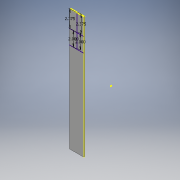
# Autodesk Inventor part: long metal piece 2x17
Saved by Autodesk Inventor 2017 (Build 210142000, 142)
## iProperties
Created: 2017-03-02
Part Number: long metal piece 2x17
Material: Generic
Document SubType Name: Modeling
Designer: Jess
Density: 1 g/cm^3
Appearance: Default
Author: Jess
Autodesk Inventor part; units mm, degrees
ref_plane "YZ Plane" through (0, 0, 0) normal (1, 0, 0) x (0, 1, 0)
ref_plane "XZ Plane" through (0, 0, 0) normal (0, 1, 0) x (-1, 0, 0)
ref_plane "XY Plane" through (0, 0, 0) normal (0, 0, 1) x (1, 0, 0)
sketch "Sketch1" plane through (0, 0, 0) normal (0, 0, 1) x (1, 0, 0)
  line L0 (-144.6628, 165.0655) -> (-93.8628, 165.0655)
  line L1 (-93.8628, 165.0655) -> (-93.8628, -263.5595)
  line L2 (-93.8628, -263.5595) -> (-144.6628, -263.5595)
  line L3 (-144.6628, -263.5595) -> (-144.6628, 165.0655)
  line L4 (-119.2628, 165.0655) -> (-119.2628, 104.7405)
  line L5 (-119.2628, 104.7405) -> (-144.6628, 104.7405)
  line L6 (-93.8628, 104.7405) -> (-119.2628, 104.7405)
  point P0 (0, 0)
  dimension "d0" = 50.8
  dimension "d1" = 428.625
  dimension "d4" = 60.325
  constraints: 14 end point, 3 perpendicular, 3 point on line, 2 parallel, 1 horizontal, 1 midpoint, 1 vertical
  measures "d0" distance of L1.end L2.end
  measures "d1" distance of L0.end L1.end
  measures "d4" distance of L4.start L4.end
extrude "Extrusion1" add sketch "Sketch1" along normal blind 3.175
sketch "Sketch2" plane through (0, 0, 3.175) normal (0, 0, 1) x (1, 0, 0)
  point P0 (0, 0)
sketch "Sketch3" plane through (0, 0, 3.175) normal (0, 0, 1) x (1, 0, 0)
  line L0 (-93.8628, 165.0655) -> (-144.6628, 165.0655) projected
  line L1 (-119.2628, 165.0655) -> (-119.2628, 104.7405)
  line L2 (-119.2628, 104.7405) -> (-144.6628, 104.7405)
  line L3 (-144.6628, 104.7405) -> (-93.8628, 104.7405)
  line L4 (-93.8628, -263.5595) -> (-93.8628, 165.0655) projected
  line L5 (-119.2628, 104.7405) -> (-119.2628, 53.9405)
  line L6 (-119.2628, 53.9405) -> (-144.6628, 53.9405)
  line L7 (-144.6628, 53.9405) -> (-93.8628, 53.9405)
  point P0 (0, 0)
  dimension "d5" = 60.325
  dimension "d7" = 50.8
  constraints: 12 end point, 4 point on line, 2 perpendicular, 2 vertical, 1 midpoint
  measures "d5" distance of L1.start L1.end
  measures "d7" distance of L1.end L5.end
sketch "Sketch4" plane through (0, 0, 0) normal (0, 0, -1) x (-1, 0, 0)
  line L0 (93.8628, 165.0655) -> (144.6628, 165.0655) projected
  line L1 (119.2628, 165.0655) -> (119.2628, 104.7405)
  line L2 (119.2628, 104.7405) -> (93.8628, 104.7405)
  line L3 (93.8628, 104.7405) -> (144.6628, 104.7405)
  line L4 (119.2628, 104.7405) -> (119.2628, 53.9405)
  line L5 (119.2628, 53.9405) -> (93.8628, 53.9405)
  line L6 (93.8628, 53.9405) -> (144.6628, 53.9405)
  point P0 (0, 0)
  dimension "d6" = 60.325
  dimension "d8" = 50.8
  constraints: 12 end point, 2 perpendicular, 2 point on line, 2 vertical, 1 midpoint
  measures "d6" distance of L1.start L1.end
  measures "d8" distance of L1.end L4.end
body "Solid1"
